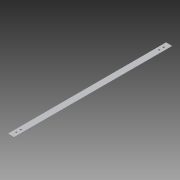
# Autodesk Inventor part: M - 26 inch rail surface
Saved by Autodesk Inventor 2013 (Build 170138000, 138)
## iProperties
Created: 2013-02-16
Part Number: M - 26 inch rail surface
Material: Aluminum 6061
Document SubType Name: Modeling
Designer: Moses
Mass: 71.5476 g
Surface Area: 355.737 cm^2
Volume: 26.4013 cm^3
Density: 2.71 g/cm^3
Author: Moses
Autodesk Inventor part; units mm, degrees
ref_plane "YZ Plane" through (0, 0, 0) normal (1, 0, 0) x (0, 1, 0)
ref_plane "XZ Plane" through (0, 0, 0) normal (0, 1, 0) x (-1, 0, 0)
ref_plane "XY Plane" through (0, 0, 0) normal (0, 0, 1) x (1, 0, 0)
sketch "Sketch1" plane through (0, 0, 0) normal (0, 1, 0) x (-1, 0, 0)
  line L0 (0, 0) -> (25.4, 0)
  line L1 (25.4, 0) -> (25.4, 660.4)
  line L2 (25.4, 660.4) -> (0, 660.4)
  line L3 (0, 660.4) -> (0, 0)
  line L4 (12.7, 660.4) -> (12.7, 0) construction
  circle A0 centre (12.7, 638.175) radius 3.3782
  circle A1 centre (12.7, 619.125) radius 3.3782
  circle A2 centre (12.7, 22.225) radius 3.3782
  circle A3 centre (12.7, 41.275) radius 3.3782
  dimension "d0" = 660.4
  dimension "d1" = 25.4
  dimension "d4" = 6.7564
  dimension "d5" = 22.225
  dimension "d6" = 19.05
  dimension "d7" = 22.225
  dimension "d8" = 19.05
  constraints: 10 end point, 4 centre point, 4 point on line, 3 equal radius, 2 midpoint, 2 parallel, 1 horizontal, 1 perpendicular
  measures "d0" distance of L2.end L0.start
  measures "d1" distance of L1.end L2.end
  measures "d4" diameter of A0
  measures "d5" distance from line of L0 A2.centre
  measures "d6" distance of A2.centre A3.centre
  measures "d7" distance from line of L2 A0.centre
  measures "d8" distance of A1.centre A0.centre
extrude "Extrusion1" add sketch "Sketch1" along normal blind 1.5875
body "Solid1"
